Supporter OLD (Autodesk Fusion 360 design; units mm, degrees)
Autodesk Fusion 360 part; units mm, degrees
sketch "Sketch1" plane through (0, 0, 0) normal (0, 1, 0) x (1, 0, 0)
  line L0 (5, 35) -> (-5, 35)
  line L1 (-5, 35) -> (-5, -35)
  line L2 (-5, -35) -> (5, -35)
  line L3 (5, -35) -> (5, 35)
  line L4 (5, 35) -> (-5, -35) construction
  line L5 (-5, 35) -> (5, -35) construction
  dimension "d1" = 10
  dimension "d2" = 70
  constraint horizontal L0
  constraint perpendicular L0 L1
  constraint parallel L0 L2
  constraint parallel L1 L3
  constraint coincident L4 origin
  constraint coincident L5 origin
  measures "d1" distance of L1.end L2.end
  measures "d2" distance of L0.end L1.end
extrude "Extrude1" add sketch "Sketch1" along normal blind 10
sketch "Sketch2" plane through (5, 0, 0) normal (1, 0, 0) x (0, 0, -1)
  line L0 (-35, 0) -> (35, 0)
  line L1 (35, 0) -> (35, 10)
  line L2 (35, 10) -> (-35, 10)
  line L3 (-35, 10) -> (-35, 0)
  circle A0 centre (0, 60) radius 3.275
  spline S0 degree 5 poles (35, 10) (34.5419, 12.294) (33.5997, 16.7974) (32.1085, 23.2982) (29.9637, 31.4555) (27.0193, 40.7815) (23.8113, 49.198) (20.344, 56.6442) (16.6298, 63.0336) (12.6921, 68.253) (8.5705, 72.156) (4.3189, 74.5848) (0, 75.4133) (-4.3189, 74.5848) (-8.5705, 72.156) (-12.6921, 68.253) (-16.6298, 63.0336) (-20.344, 56.6442) (-23.8113, 49.198) (-27.0193, 40.7815) (-29.9637, 31.4555) (-32.1085, 23.2982) (-33.5997, 16.7974) (-34.5419, 12.294) (-35, 10) knots 0 0 0 0 0 0 0.05 0.1 0.15 0.2 0.25 0.3 0.35 0.4 0.45 0.5 0.55 0.6 0.65 0.7 0.75 0.8 0.85 0.9 0.95 1 1 1 1 1 1
  point P0 (15, 65)
  point P1 (0, 75)
  point P2 (-15, 65)
  dimension "d8" = 6.55
  dimension "d16" = 50
  dimension "d17" = 35
  constraint coincident L1.end L2.start
  constraint coincident L2.end L3.start
  measures "d8" diameter of A0
  measures "d16" distance of L2 A0.centre
  measures "d17" distance of L3 A0.centre
extrude "Extrude3" add sketch "Sketch2" against normal blind 10 contours L2 S0
